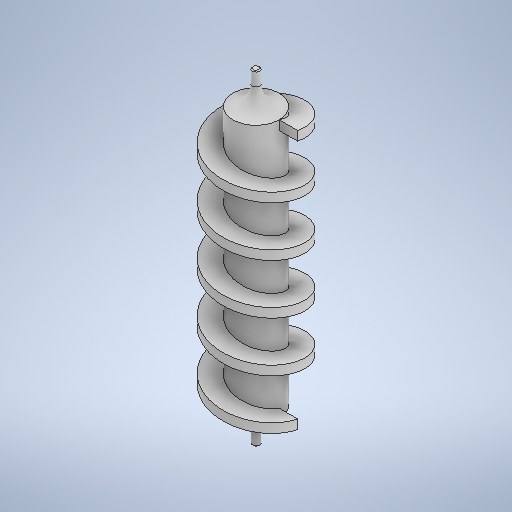
# Autodesk Inventor part: Archimedes Screw
Saved by Autodesk Inventor 2025.3 (Build 293356000, 356)
## iProperties
Created: 2026-03-08
Part Number: Archimedes Screw
Material: Generic
Document SubType Name: Modeling
Designer: ziada
Density: 1 g/cm^3
Appearance: Default
Mass: 893.601 g
Surface Area: 1049.58 cm^2
Volume: 893.601 cm^3
Author: ziada
## iProperties of the stored document Archimedes Screw V2_3DPrint.ipt
Created: 2026-04-11
Part Number: Archimedes Screw V2_3DPrint
Material: Generic
Document SubType Name: Modeling
Designer: ziada
Density: 1 g/cm^3
Appearance: Default
Author: ziada
Autodesk Inventor part; units mm, degrees
ref_plane "YZ Plane" through (0, 0, 0) normal (1, 0, 0) x (0, 1, 0)
ref_plane "XZ Plane" through (0, 0, 0) normal (0, 1, 0) x (-1, 0, 0)
ref_plane "XY Plane" through (0, 0, 0) normal (0, 0, 1) x (1, 0, 0)
sketch "Sketch1" plane through (0, 0, 0) normal (0, 1, 0) x (-1, 0, 0)
  circle A0 centre (0, 0) radius 25
  dimension "d0" = 50
  constraints: 1 centre point, 1 coincident
  measures "d0" diameter of A0
extrude "Extrusion1" add sketch "Sketch1" along normal blind 280
sketch "Sketch2" plane through (0, 0, 0) normal (0, 0, 1) x (1, 0, 0)
  line L0 (25, 0) -> (-25, 0) projected
  line L1 (0, 0) -> (0, 300)
  line L2 (45, 0) -> (45, 10)
  line L3 (45, 10) -> (20, 10)
  line L4 (20, 10) -> (20, 0)
  line L5 (45, 0) -> (20, 0)
  dimension "d5" = 300
  dimension "d26" = 25
  dimension "d27" = 10
  constraints: 10 end point, 1 collinear, 1 horizontal, 1 midpoint, 1 perpendicular, 1 point on line, 1 vertical
  measures "d5" distance of L1.start L1.end
  measures "d26" distance of L2.end L3.end
  measures "d27" distance of L2.start L2.end
coil "Coil1" sketch "Sketch2" operation add axis through (0, -10, 0) along (0, 1, 0) pitch 54 turns 5 hand left
sketch "Sketch3" plane through (0, 0, 0) normal (0, -1, 0) x (1, 0, 0)
  circle A0 centre (0, 0) radius 4
  dimension "d16" = 8
  constraints: 1 centre point, 1 coincident
  measures "d16" diameter of A0
extrude "Extrusion2" add sketch "Sketch3" along normal blind 36
fillet "Fillet1" radius 21 1 edges at (-4, 0, 0)
sketch "Sketch4" plane through (0, 280, 0) normal (0, 1, 0) x (1, 0, 0)
  circle A0 centre (0, 0) radius 4 projected
  circle A1 centre (0, 0) radius 4
  dimension "d20" = 8
  constraints: 1 centre point, 1 coincident
  measures "d20" diameter of A1
extrude "Extrusion3" add sketch "Sketch4" along normal blind 36
fillet "Fillet2" radius 21 1 edges at (-4, 280, 0)
chamfer "Chamfer1" distance 1 angle 45 2 edges at (-4, 316, 0) (-4, -36, 0)
body "Solid1"
